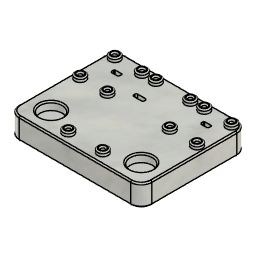
Remote (Autodesk Fusion 360 design; units mm, degrees)
Autodesk Fusion 360 part; units mm, degrees
sketch "Sketch1" plane through (0, 0, 0) normal (0, 0, 1) x (1, 0, 0)
  line L0 (-42, 40) -> (42, 40)
  line L1 (50, 32) -> (50, -32)
  line L2 (42, -40) -> (-42, -40)
  line L3 (-50, -32) -> (-50, 32)
  line L4 (0, 40) -> (0, -40) construction
  arc A0 (-42, 40) -> (-50, 32) centre (-42, 32) ccw
  arc A1 (50, 32) -> (42, 40) centre (42, 32) ccw
  arc A2 (-50, -32) -> (-42, -40) centre (-42, -32) ccw
  arc A3 (42, -40) -> (50, -32) centre (42, -32) ccw
  circle A4 centre (-44, 34) radius 1.4
  circle A5 centre (-23.5, 34) radius 1.4
  circle A6 centre (-23.5, 8) radius 1.4
  circle A7 centre (-44, 8) radius 1.4
  circle A8 centre (-13, 34) radius 1.4
  circle A9 centre (-13, -32) radius 1.4
  circle A10 centre (-34, -24) radius 8.35
  circle A11 centre (-44, 34) radius 4
  circle A12 centre (-23.5, 34) radius 4
  circle A13 centre (-13, 34) radius 4
  circle A14 centre (-23.5, 8) radius 4
  circle A15 centre (-44, 8) radius 4
  circle A16 centre (-13, -32) radius 4
  circle A17 centre (-38.75, 33) radius 1.6
  circle A18 centre (-28.75, 33) radius 1.6
  circle A19 centre (13, 34) radius 1.4
  circle A20 centre (13, 34) radius 4
  circle A21 centre (23.5, 34) radius 4
  circle A22 centre (23.5, 34) radius 1.4
  circle A23 centre (28.75, 33) radius 1.6
  circle A24 centre (38.75, 33) radius 1.6
  circle A25 centre (44, 34) radius 1.4
  circle A26 centre (44, 34) radius 4
  circle A27 centre (44, 8) radius 4
  circle A28 centre (44, 8) radius 1.4
  circle A29 centre (23.5, 8) radius 1.4
  circle A30 centre (23.5, 8) radius 4
  circle A31 centre (34, -24) radius 8.35
  circle A32 centre (13, -32) radius 4
  circle A33 centre (13, -32) radius 1.4
  point P0 (-50, 40)
  point P1 (50, 40)
  point P2 (-50, -40)
  dimension "d1" = 100
  dimension "d2" = 80
  dimension "d3" = 8
  dimension "d4" = 8
  dimension "d5" = 8
  dimension "d6" = 2.8
  dimension "d8" = 2.8
  dimension "d9" = 20.5
  dimension "d12" = 2.8
  dimension "d13" = 2.8
  dimension "d14" = 26
  dimension "d15" = 6
  dimension "d16" = 6
  dimension "d17" = 2.8
  dimension "d18" = 10.5
  dimension "d19" = 2.8
  dimension "d20" = 66
  dimension "d21" = 16.7
  dimension "d22" = 16
  dimension "d23" = 16
  dimension "d24" = 8
  dimension "d25" = 8
  dimension "d26" = 8
  dimension "d27" = 8
  dimension "d28" = 8
  dimension "d29" = 8
  dimension "d30" = 3.2
  dimension "d31" = 3.2
  dimension "d32" = 7
  dimension "d33" = 10
  dimension "d34" = 5.25
  constraint horizontal L0
  constraint vertical L1
  constraint horizontal L2
  constraint vertical L3
  constraint midpoint origin L4
  constraint coincident L0 L4.start
  constraint coincident P0 L0
  constraint coincident P0 L3
  constraint tangent L0 A0
  constraint tangent L3 A0
  constraint coincident P1 L0
  constraint coincident P1 L1
  constraint tangent L0 A1
  constraint tangent L1 A1
  constraint coincident L2 L4.end
  constraint coincident P2 L2
  constraint coincident P2 L3
  constraint tangent L2 A2
  constraint tangent L3 A2
  constraint tangent L1 A3
  constraint tangent L2 A3
  constraint equal A2 A3
  constraint vertical A5.centre A6.centre
  constraint horizontal A7.centre A6.centre
  constraint horizontal A4.centre A5.centre
  constraint midpoint L0 L4.start
  constraint midpoint L2 L4.end
  constraint vertical A4.centre A7.centre
  constraint horizontal A5.centre A8.centre
  constraint vertical A8.centre A9.centre
  constraint concentric A4 A11
  constraint concentric A5 A12
  constraint concentric A8 A13
  constraint concentric A6 A14
  constraint concentric A7 A15
  constraint concentric A9 A16
  constraint horizontal A17.centre A18.centre
  constraint symmetric L4 A4 A25
  constraint symmetric L4 A5 A22
  constraint symmetric L4 A6 A29
  constraint symmetric L4 A7 A28
  constraint symmetric L4 A8 A19
  constraint symmetric L4 A10 A31
  constraint symmetric L4 A11 A26
  constraint symmetric L4 A12 A21
  constraint symmetric L4 A13 A20
  constraint symmetric L4 A14 A30
  constraint symmetric L4 A15 A27
  constraint symmetric L4 A17 A24
  constraint symmetric L4 A18 A23
  constraint symmetric L4 A9 A33
  constraint symmetric L4 A16 A32
  measures "d1" distance of P0 P1
  measures "d2" distance of P0 P2
  measures "d3" radius of A0
  measures "d4" radius of A1
  measures "d5" radius of A2
  measures "d6" diameter of A4
  measures "d8" diameter of A5
  measures "d9" distance of A4.centre A5.centre
  measures "d12" diameter of A7
  measures "d13" diameter of A6
  measures "d14" distance of A4.centre A7.centre
  measures "d15" distance of L3 A7.centre
  measures "d16" distance of L0 A5.centre
  measures "d17" diameter of A8
  measures "d18" distance of A5.centre A8.centre
  measures "d19" diameter of A9
  measures "d20" distance of A8.centre A9.centre
  measures "d21" diameter of A10
  measures "d22" distance of L2 A10.centre
  measures "d23" distance of L3 A10.centre
  measures "d24" diameter of A11
  measures "d25" diameter of A12
  measures "d26" diameter of A13
  measures "d27" diameter of A14
  measures "d28" diameter of A15
  measures "d29" diameter of A16
  measures "d30" diameter of A17
  measures "d31" diameter of A18
  measures "d32" distance of L0 A17.centre
  measures "d33" distance of A17.centre A18.centre
  measures "d34" horizontal distance of A4.centre A17.centre
extrude "Extrude1" add sketch "Sketch1" along normal blind 16 contours L0 L1 L2 L3 A0 A1 A2 A3 | A11 A17 | A12 A18 | A21 A23 | A24 A26 picked at (-39.1081, 33.0896) picked at (-28.3883, 33.0689) picked at (28.3919, 33.0896) picked at (39.1117, 33.0689)
extrude "Extrude2" add sketch "Sketch1" along normal blind 19 contours A11 A17 | A11 A17 | A12 A18 | A12 A18 | A13 | A14 | A15 | A16 | A20 | A21 A23 | A21 A23 | A24 A26 | A24 A26 | A27 | A30 | A32 picked at (-40.9283, 34.2047) picked at (-40.1512, 33.3052) picked at (-26.2957, 32.7469) picked at (-27.3359, 33.2404) picked at (26.5717, 34.2047) picked at (27.3488, 33.3052) picked at (40.1641, 33.2404) picked at (41.2043, 32.7469)
extrude "Extrude3" add sketch "Sketch1" along normal blind 13 contours A4 | A5 | A6 | A7 | A8 | A9 | A19 | A22 | A25 | A28 | A29 | A33
extrude "Extrude5" add sketch "Sketch1" along normal blind 10 contours A10 | A31
sketch "Sketch2" plane through (0, 0, 0) normal (0, 0, 1) x (1, 0, 0)
  line L0 (23.75, 16.25) -> (-23.75, 16.25)
  line L1 (-24.75, 15.25) -> (-24.75, -35.25)
  line L2 (-23.75, -36.25) -> (23.75, -36.25)
  line L3 (24.75, -35.25) -> (24.75, 15.25)
  arc A0 (24.75, 15.25) -> (23.75, 16.25) centre (23.75, 15.25) ccw
  arc A1 (-23.75, 16.25) -> (-24.75, 15.25) centre (-23.75, 15.25) ccw
  arc A2 (-24.75, -35.25) -> (-23.75, -36.25) centre (-23.75, -35.25) ccw
  arc A3 (23.75, -36.25) -> (24.75, -35.25) centre (23.75, -35.25) ccw
  line L4 (24.75, -10) -> (-24.75, -10) construction
  line L5 (0, 0) -> (0, -10) construction
  point P0 (24.75, 16.25)
  point P1 (-24.75, 16.25)
  point P2 (24.75, -36.25)
  point P3 (-8.75, 13.25)
  dimension "d41" = 49.5
  dimension "d42" = 52.5
  dimension "d43" = 1
  dimension "d73" = 10
  constraint horizontal L0
  constraint vertical L1
  constraint horizontal L2
  constraint vertical L3
  constraint coincident P0 L0
  constraint coincident P0 L3
  constraint tangent L0 A0
  constraint tangent L3 A0
  constraint coincident P1 L0
  constraint coincident P1 L1
  constraint tangent L0 A1
  constraint tangent L1 A1
  constraint equal A0 A1
  constraint tangent L1 A2
  constraint tangent L2 A2
  constraint equal A0 A2
  constraint coincident P2 L2
  constraint coincident P2 L3
  constraint tangent L2 A3
  constraint tangent L3 A3
  constraint equal A0 A3
  constraint midpoint L3 L4.start
  constraint midpoint L1 L4.end
  constraint coincident L5.start origin
  constraint midpoint L4 L5.end
  constraint vertical L5
  measures "d41" distance of P0 P1
  measures "d42" distance of P0 P2
  measures "d43" radius of A0
  measures "d73" distance of L5.start L5.end
extrude "Extrude4" cut sketch "Sketch2" along normal blind 12.5
sketch "Sketch3" plane through (0, 40, 0) normal (0, 1, 0) x (-1, 0, 0)
  line L0 (-42, 0) -> (42, 0)
  line L1 (42, 0) -> (42, 16)
  line L2 (42, 16) -> (-42, 16)
  line L3 (-42, 16) -> (-42, 0)
ref_plane "WorkPlane1" through (0, 0, 8) normal (0, 0, -1) x (-1, 0, 0)
sketch "Sketch4" plane through (0, 0, 8) normal (0, 0, -1) x (-1, 0, 0)
  line L0 (0, 40) -> (0, -40) construction
  line L1 (-43.85, 40) -> (-23.65, 40)
  line L2 (-23.65, 40) -> (-23.65, 29.5)
  line L3 (-23.65, 29.5) -> (-43.85, 29.5)
  line L4 (-43.85, 29.5) -> (-43.85, 40)
  line L5 (-50, -32) -> (-50, 32)
  line L6 (-42.25, 29.5) -> (-25.25, 29.5)
  line L7 (-25.25, 29.5) -> (-25.25, 25.5)
  line L8 (-27.25, 23.5) -> (-40.25, 23.5)
  line L9 (-42.25, 25.5) -> (-42.25, 29.5)
  arc A0 (-27.25, 23.5) -> (-25.25, 25.5) centre (-27.25, 25.5) ccw
  arc A1 (-42.25, 25.5) -> (-40.25, 23.5) centre (-40.25, 25.5) ccw
  line L10 (-42, 40) -> (42, 40)
  line L11 (-36.75, 23.5) -> (-30.75, 23.5)
  line L12 (-30.75, 23.5) -> (-30.75, 26)
  line L13 (-31.25, 26.5) -> (-36.25, 26.5)
  line L14 (-36.75, 26) -> (-36.75, 23.5)
  arc A2 (-36.25, 26.5) -> (-36.75, 26) centre (-36.25, 26) ccw
  arc A3 (-30.75, 26) -> (-31.25, 26.5) centre (-31.25, 26) ccw
  line L15 (6.5, 40) -> (-6.5, 40)
  line L16 (-6.5, 40) -> (-6.5, 22)
  line L17 (-6.5, 22) -> (6.5, 22)
  line L18 (6.5, 22) -> (6.5, 40)
  line L19 (5, 22) -> (-5, 22)
  line L20 (-5, 22) -> (-5, 16.25)
  line L21 (-5, 16.25) -> (5, 16.25)
  line L22 (5, 16.25) -> (5, 22)
  line L23 (-23.75, 16.25) -> (23.75, 16.25)
  line L24 (5, 16.25) -> (13, 16.25)
  line L25 (13, 16.25) -> (13, 19.25)
  line L26 (13, 19.25) -> (5, 19.25)
  line L27 (5, 19.25) -> (5, 16.25)
  point P0 (-42.25, 23.5)
  point P1 (-36.75, 26.5)
  dimension "d55" = 20.2
  dimension "d56" = 10.5
  dimension "d57" = 6.15
  dimension "d58" = 17
  dimension "d59" = 6
  dimension "d60" = 2
  dimension "d61" = 6
  dimension "d62" = 3
  dimension "d63" = 0.5
  dimension "d74" = 13
  dimension "d75" = 18
  dimension "d76" = 10
  dimension "d79" = 8
  dimension "d80" = 3
  constraint vertical L0
  constraint horizontal L1
  constraint vertical L2
  constraint horizontal L3
  constraint vertical L4
  constraint horizontal L6
  constraint vertical L7
  constraint horizontal L8
  constraint vertical L9
  constraint coincident L3 L6.start
  constraint midpoint L3 L6
  constraint tangent L7 A0
  constraint tangent L8 A0
  constraint coincident P0 L8
  constraint coincident P0 L9
  constraint tangent L8 A1
  constraint tangent L9 A1
  constraint equal A0 A1
  constraint collinear L1 L10
  constraint horizontal L11
  constraint vertical L12
  constraint horizontal L13
  constraint vertical L14
  constraint coincident L8 L11.start
  constraint midpoint L8 L11
  constraint coincident P1 L13
  constraint coincident P1 L14
  constraint tangent L13 A2
  constraint tangent L14 A2
  constraint tangent L12 A3
  constraint tangent L13 A3
  constraint equal A2 A3
  constraint horizontal L15
  constraint vertical L16
  constraint horizontal L17
  constraint vertical L18
  constraint coincident L10 L15.start
  constraint midpoint L10 L15
  constraint horizontal L19
  constraint vertical L20
  constraint horizontal L21
  constraint vertical L22
  constraint coincident L17 L19.start
  constraint midpoint L17 L19
  constraint collinear L21 L23
  constraint horizontal L24
  constraint vertical L25
  constraint horizontal L26
  constraint vertical L27
  measures "d55" distance of L1.start L1.end
  measures "d56" distance of L1.end L2.end
  measures "d57" distance of L4 L5
  measures "d58" distance of L6.start L6.end
  measures "d59" distance of L6.start P0
  measures "d60" radius of A0
  measures "d61" distance of L11.start L11.end
  measures "d62" distance of L11.start P1
  measures "d63" radius of A2
  measures "d74" distance of L15.start L15.end
  measures "d75" distance of L15.start L17.end
  measures "d76" distance of L20.end L21.end
  measures "d79" distance of L21.end L24.end
  measures "d80" distance of L21.end L26.end
extrude "Extrude7" cut sketch "Sketch4" along normal mid plane 6.6 contours L1 L2 L3 L4 L6 L10 | L3 L6 L7 L8 L9 A0 A1 L12 L13 L14 A2 A3 | L8 L11 L12 L13 L14 A2 A3
extrude "Extrude8" cut sketch "Sketch4" against normal blind 8 contours L8 L11 L12 L13 L14 A2 A3
extrude "Extrude9" cut sketch "Sketch4" along normal mid plane 13.2 contours L10 L15 L16 L17 L18 L19 | L17 L19 L20 L21 L22 L23 L27
extrude "Extrude10" cut sketch "Sketch4" against normal blind 21 contours L22 L23 L24 L25 L26 L27
mirror "Mirror1" about plane through (0, 0, 0) normal (1, 0, 0) of "Extrude7", "Extrude8"
fillet "Fillet1" radius 1 56 edges at (9.2707, -33.4465, 19) (11.6947, -31.4937, 19) (-14.3053, -31.4937, 19) (-16.7293, -33.4465, 19) (19.7707, 6.5535, 19) (22.1947, 8.5063, 19) (40.2707, 6.5535, 19) (42.6947, 8.5063, 19) (22.1947, 34.5063, 19) (19.7707, 32.5535, 19) (42.6947, 34.5063, 19) (40.2707, 32.5535, 19) (30.75, 23.5, 13.65) (36.75, 23.5, 13.65) (-14.3053, 34.5063, 19) (-16.7293, 32.5535, 19) (-24.8053, 34.5063, 19) (-27.2293, 32.5535, 19) (-24.8053, 8.5063, 19) (-27.2293, 6.5535, 19) (-45.3053, 8.5063, 19) (-47.7293, 6.5535, 19) (-45.3053, 34.5063, 19) (-47.7293, 32.5535, 19) (-36.75, 23.5, 13.65) (-30.75, 23.5, 13.65) (11.6947, 34.5063, 19) (9.2707, 32.5535, 19) (-24.75, -10, 0) (-24.4571, -35.9571, 0) (0, -36.25, 0) (24.4571, -35.9571, 0) (24.75, -10, 0) (24.4571, 15.9571, 0) (0, 16.25, 0) (-24.4571, 15.9571, 0) (47.6569, -37.6569, 0) (50, 0, 0) (47.6569, 37.6569, 0) (0, 40, 0) (-47.6569, 37.6569, 0) (-50, 0, 0) (-47.6569, -37.6569, 0) (0, -40, 0) (0, 40, 16) (-47.6569, 37.6569, 16) (-50, 0, 16) (-47.6569, -37.6569, 16) (0, -40, 16) (47.6569, -37.6569, 16) (50, 0, 16) (47.6569, 37.6569, 16) (-13, 19.25, 12) (-13, 16.25, 14.25) (-5, 19.25, 15.3) (-5, 16.25, 15.3)
chamfer "Chamfer1" distance 1 angle 45 2 edges at (-41.7849, -20.9805, 16) (26.2151, -20.9805, 16)
equation "d34 = ( ( 20.5 - 10 ) / 2 ) * 1 mm"
equation "d57 = 16.25 mm - 10.1 mm"
